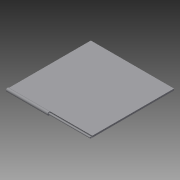
# Autodesk Inventor part: zawias2
Saved by Autodesk Inventor 2014 (Build 180170000, 170)
## iProperties
Created: 2013-12-27
Part Number: zawias2
Material: Ogólny
Document SubType Name: Modeling
Designer: Kuba
Density: 1 g/cm^3
Appearance: Domyślna
Author: Kuba
Autodesk Inventor part; units mm, degrees
ref_plane "YZ Plane" through (0, 0, 0) normal (1, 0, 0) x (0, 1, 0)
ref_plane "XZ Plane" through (0, 0, 0) normal (0, 1, 0) x (-1, 0, 0)
ref_plane "XY Plane" through (0, 0, 0) normal (0, 0, 1) x (1, 0, 0)
sketch "Szkic1" plane through (0, 0, 0) normal (1, 0, 0) x (0, 1, 0)
  line L0 (0, 0) -> (-49.134, 0)
  line L1 (-49.134, 1) -> (0, 1)
  line L2 (0, 1) -> (0, 0)
  circle A0 centre (-50, 0.5) radius 1
  circle A1 centre (-50, 0.5) radius 0.5
  dimension "d0" = 2
  dimension "d1" = 1
  dimension "d2" = 49.134
  dimension "d3" = 1
  constraints: 6 end point, 2 centre point, 2 point on circle, 1 coincident, 1 horizontal, 1 parallel
  measures "d0" diameter of A0
  measures "d1" distance of L1.end L0.start
  measures "d2" distance of L1.start L1.end
  measures "d3" diameter of A1
extrude "Wyciągnięcie proste1" add sketch "Szkic1" along normal blind 50 contours L0 A0 L1 L2
extrude "Wyciągnięcie proste2" add sketch "Szkic1" along normal blind 50 contours A1
extrude "Wyciągnięcie proste3" add sketch "Szkic1" along normal blind 25 contours A0
